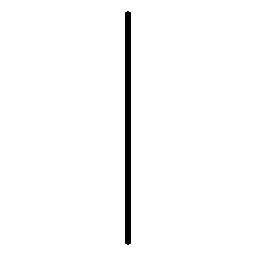
2020 V slot v1 (Autodesk Fusion 360 design; units mm, degrees)
Autodesk Fusion 360 part; units mm, degrees
sketch "Sketch1" plane through (0, 0, 0) normal (0, 0, 1) x (1, 0, 0)
  circle A0 centre (0, 0) radius 2.15
  line L0 (3.75, 2.8308) -> (3.75, -2.8308)
  line L1 (8.2, -3.1) -> (10, -4.9)
  line L2 (10, -4.9) -> (10, -10)
  line L3 (-2.8308, 3.75) -> (2.8308, 3.75)
  line L4 (-3.75, -2.8308) -> (-3.75, 2.8308)
  line L5 (2.8308, -3.75) -> (-2.8308, -3.75)
  line L6 (6.1096, -5.1904) -> (8.2, -5.1904)
  line L7 (8.2, -5.1904) -> (8.2, -3.1)
  line L8 (6.1096, -5.1904) -> (3.75, -2.8308)
  line L9 (10, -10) -> (4.9, -10)
  line L10 (4.9, -10) -> (3.1, -8.2)
  line L11 (3.1, -8.2) -> (5.1904, -8.2)
  line L12 (5.1904, -8.2) -> (5.1904, -6.1096)
  line L13 (5.1904, -6.1096) -> (2.8308, -3.75)
  line L14 (8.2, 3.1) -> (8.2, 5.1904)
  line L15 (10, 10) -> (10, 4.9)
  line L16 (8.2, 5.1904) -> (6.1096, 5.1904)
  line L17 (5.1904, 8.2) -> (3.1, 8.2)
  line L18 (6.1096, 5.1904) -> (3.75, 2.8308)
  line L19 (5.1904, 6.1096) -> (5.1904, 8.2)
  line L20 (4.9, 10) -> (10, 10)
  line L21 (10, 4.9) -> (8.2, 3.1)
  line L22 (5.1904, 6.1096) -> (2.8308, 3.75)
  line L23 (3.1, 8.2) -> (4.9, 10)
  line L24 (-3.1, 8.2) -> (-5.1904, 8.2)
  line L25 (-10, 10) -> (-4.9, 10)
  line L26 (-5.1904, 8.2) -> (-5.1904, 6.1096)
  line L27 (-8.2, 5.1904) -> (-8.2, 3.1)
  line L28 (-5.1904, 6.1096) -> (-2.8308, 3.75)
  line L29 (-6.1096, 5.1904) -> (-8.2, 5.1904)
  line L30 (-10, 4.9) -> (-10, 10)
  line L31 (-4.9, 10) -> (-3.1, 8.2)
  line L32 (-6.1096, 5.1904) -> (-3.75, 2.8308)
  line L33 (-8.2, 3.1) -> (-10, 4.9)
  line L34 (-8.2, -3.1) -> (-8.2, -5.1904)
  line L35 (-10, -10) -> (-10, -4.9)
  line L36 (-8.2, -5.1904) -> (-6.1096, -5.1904)
  line L37 (-5.1904, -8.2) -> (-3.1, -8.2)
  line L38 (-6.1096, -5.1904) -> (-3.75, -2.8308)
  line L39 (-5.1904, -6.1096) -> (-5.1904, -8.2)
  line L40 (-4.9, -10) -> (-10, -10)
  line L41 (-10, -4.9) -> (-8.2, -3.1)
  line L42 (-5.1904, -6.1096) -> (-2.8308, -3.75)
  line L43 (-3.1, -8.2) -> (-4.9, -10)
  dimension "d24" = 4.3
  dimension "d39" = 360
  dimension "d45" = 360
  constraint coincident A0.centre origin
  constraint perpendicular L11 L12
  measures "d24" diameter of A0
extrude "Extrude1" add sketch "Sketch1" along normal blind 1500
fillet "Fillet1" radius 0.3 4 edges at (-10, -10, 750) (-10, 10, 750) (10, -10, 750) (10, 10, 750)
fillet "Fillet2" radius 0.3 8 edges at (3.1, 8.2, 750) (-3.1, 8.2, 750) (-8.2, -3.1, 750) (3.1, -8.2, 750) (8.2, -3.1, 750) (-3.1, -8.2, 750) (8.2, 3.1, 750) (-8.2, 3.1, 750)
fillet "Fillet3" radius 0.3 8 edges at (8.2, 5.1904, 750) (5.1904, 8.2, 750) (8.2, -5.1904, 750) (5.1904, -8.2, 750) (-5.1904, -8.2, 750) (-8.2, -5.1904, 750) (-8.2, 5.1904, 750) (-5.1904, 8.2, 750)
